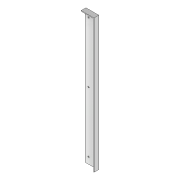
# Autodesk Inventor part: Guias de bandeja 2
Saved by Autodesk Inventor 2020.3 (Build 243373000, 373)
## iProperties
Created: 2020-05-08
Part Number: Guias de bandeja 2
Material: Aluminum 1100-H14
Document SubType Name: Modeling
Designer: Pipi
Density: 2.7 g/cm^3
Appearance: Satin
Author: Pipi
Autodesk Inventor part; units mm, degrees
ref_plane "YZ Plane" through (0, 0, 0) normal (1, 0, 0) x (0, 1, 0)
ref_plane "XZ Plane" through (0, 0, 0) normal (0, 1, 0) x (-1, 0, 0)
ref_plane "XY Plane" through (0, 0, 0) normal (0, 0, 1) x (1, 0, 0)
sketch "Boceto1" plane through (0, 0, 0) normal (0, 1, 0) x (-1, 0, 0)
  line L0 (30.8526, 17.8417) -> (30.8526, 15.8417)
  line L1 (30.8526, 15.8417) -> (-9.1474, 15.8417)
  line L2 (-9.1474, 15.8417) -> (-9.1474, 30.8417)
  line L3 (-9.1474, 30.8417) -> (-7.1474, 30.8417)
  line L4 (-7.1474, 30.8417) -> (-7.1474, 17.8417)
  line L5 (-7.1474, 17.8417) -> (30.8526, 17.8417)
  dimension "d0" = 2
  dimension "d1" = 40
  dimension "d2" = 15
  dimension "d3" = 2
  constraints: 12 end point, 5 perpendicular, 1 vertical
  measures "d0" distance of L0.start L0.end
  measures "d1" distance of L0.end L1.end
  measures "d2" distance of L1.end L2.end
  measures "d3" distance of L2.end L3.end
extrude "Extrusión1" add sketch "Boceto1" along normal blind 414
sketch "Boceto5" plane through (-30.8526, 0, 17.8417) normal (0, 0, 1) x (1, 0, 0)
  line L0 (38, 0) -> (40, 0) projected
  line L1 (40, 0) -> (10, 0)
  line L2 (0, 0) -> (38, 0) projected
  line L3 (10, 0) -> (10, 414)
  line L4 (10, 414) -> (34, 414)
  line L5 (0, 414) -> (38, 414) projected
  circle A0 centre (10, 394) radius 2
  circle A1 centre (10, 207) radius 2
  circle A2 centre (10, 20) radius 2
  point P0 (30.8526, 0)
  dimension "d21" = 30
  dimension "d22" = 414
  dimension "d23" = 4
  dimension "d24" = 4
  dimension "d25" = 4
  dimension "d26" = 20
  dimension "d27" = 207
  dimension "d28" = 20
  constraints: 6 end point, 3 centre point, 3 point on line, 1 collinear, 1 midpoint, 1 perpendicular
  measures "d21" distance of L0.end L1.end
  measures "d22" distance of L1.end L3.end
  measures "d23" diameter of A0
  measures "d24" diameter of A1
  measures "d25" diameter of A2
  measures "d26" distance from line of L2 A2.centre
  measures "d27" distance from line of L1 A1.centre
  measures "d28" distance of L3.end A0.centre
sketch "Boceto6" plane through (0, 414, 0) normal (0, 1, 0) x (1, 0, 0)
  line L0 (7.1474, -17.8417) -> (7.1474, -30.8417) projected
  line L1 (7.1474, -30.8417) -> (-30.8526, -30.8417)
  line L2 (-30.8526, -17.8417) -> (7.1474, -17.8417) projected
  line L3 (-30.8526, -30.8417) -> (-30.8526, -17.8417)
  point P0 (0, 0)
  constraints: 4 end point, 1 horizontal, 1 perpendicular
extrude "Extrusión4" add sketch "Boceto6" against normal blind 2
extrude "Extrusión5" cut sketch "Boceto5" against normal blind 2
